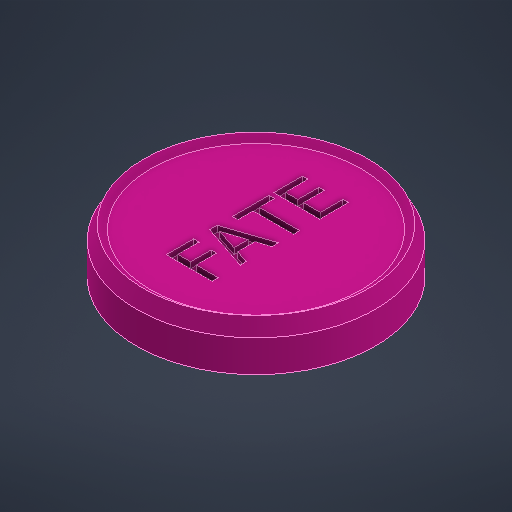
# Autodesk Inventor part: Fate Game Piece V1.01
Saved by Autodesk Inventor 2027 (Build 310192000, 192)
## iProperties
Created: 2025-10-12
Part Number: Fate Game Piece V1.01
Material: Generic
Document SubType Name: Modeling
Designer: Owner
Density: 1 g/cm^3
Appearance: Default
Author: Owner
Autodesk Inventor part; units mm, degrees
ref_plane "YZ Plane" through (0, 0, 0) normal (1, 0, 0) x (0, 1, 0)
ref_plane "XZ Plane" through (0, 0, 0) normal (0, 1, 0) x (-1, 0, 0)
ref_plane "XY Plane" through (0, 0, 0) normal (0, 0, 1) x (1, 0, 0)
sketch "Sketch1" plane through (0, 0, 0) normal (0, 0, 1) x (1, 0, 0)
  line L0 (-15.875, 0) -> (0, 0)
  line L1 (0, 0) -> (0, -4.2333)
  line L2 (0, -4.2333) -> (-15.875, -4.2333)
  line L3 (-15.875, -4.2333) -> (-15.875, 0)
  line L4 (0, -4.2333) -> (-13.97, -4.2333)
  line L5 (-13.97, -4.2333) -> (-13.97, -5.5033)
  line L6 (-13.97, -5.5033) -> (0, -5.5033)
  line L7 (0, -5.5033) -> (0, -4.2333)
  line L8 (-15.875, -4.2333) -> (-13.6299, -4.2333) construction
  line L9 (-15.875, 0) -> (-12.7, 0) construction
  line L10 (-13.97, 1.27) -> (0, 1.27)
  line L11 (0, 1.27) -> (0, 0)
  line L12 (0, 0) -> (-13.97, 0)
  line L13 (-13.97, 0) -> (-13.97, 1.27)
  line L14 (-15.875, 0) -> (-12.8362, 0) construction
  line L15 (-15.875, -4.2333) -> (-13.97, -5.5033)
  line L16 (-15.875, 0) -> (-14.9225, 1.905)
  line L17 (-14.9225, 1.905) -> (-13.97, 1.27)
  line L18 (-13.97, 0) -> (-15.875, 0)
  line L19 (0, -6.985) -> (0, 3.3867) projected
  point P0 (0, 0)
  point P1 (-13.97, 0.635)
  point P2 (0, 0.635)
  point P3 (-6.985, -4.2333)
  point P4 (-14.9225, 0)
  dimension "d0" = 0
  dimension "d1" = 4.2333
  dimension "d2" = 15.875
  dimension "d3" = 0
  dimension "d5" = 13.97
  dimension "d9" = 13.97
  dimension "d10" = 1.27
  dimension "d11" = 1.27
  dimension "d12" = 0.635
  dimension "d13" = 0
  constraints: 38 end point, 6 horizontal, 6 parallel, 4 midpoint, 3 perpendicular, 1 collinear
  measures "d0" distance from line of point (0, 0) L1
  measures "d1" distance between parallel lines of L2 L0
  measures "d2" distance of L1.end L2.end
  measures "d3" distance from line of point (0, 0) L0
  measures "d5" distance between parallel lines of L7 L5
  measures "d9" distance of point (-13.97, 0.635) point (0, 0.635)
  measures "d10" distance from line of L6 point (-6.985, -4.233)
  measures "d11" distance between parallel lines of L0 L10
  measures "d12" distance from line of L10 L16.end
  measures "d13" horizontal distance of L16.end point (-14.923, 0)
revolve "Revolution1" add sketch "Sketch1" angle 360 about axis through (0, -10, 0) along (0, 1, 0)
sketch "Sketch2" plane through (0, 1.27, 0) normal (0, 1, 0) x (1, 0, 0)
  line L0 (-2.3268, -5.2364) -> (-2.3268, -8.072)
  line L1 (-2.3268, -8.072) -> (-0.6076, -8.072)
  line L2 (-0.6076, -8.072) -> (-0.6076, -5.355)
  line L3 (-0.6076, -5.355) -> (0.1136, -5.355)
  line L4 (0.1136, -5.355) -> (0.1136, -8.072)
  line L5 (0.1136, -8.072) -> (3.048, -8.072)
  line L6 (3.048, -8.072) -> (3.048, -8.8822)
  line L7 (3.048, -8.8822) -> (-3.048, -8.8822)
  line L8 (-3.048, -8.8822) -> (-3.048, -5.2364)
  line L9 (-3.048, -5.2364) -> (-2.3268, -5.2364)
  line L10 (3.048, -5.1673) -> (-3.048, -3.1122)
  line L11 (-3.048, -3.1122) -> (-3.048, -2.1143)
  line L12 (-3.048, -2.1143) -> (3.048, -0.0593)
  line L13 (3.048, -0.0593) -> (3.048, -0.9139)
  line L14 (3.048, -0.9139) -> (1.3437, -1.4672)
  line L15 (1.3437, -1.4672) -> (1.3437, -3.7939)
  line L16 (1.3437, -3.7939) -> (3.048, -4.3472)
  line L17 (3.048, -4.3472) -> (3.048, -5.1673)
  line L18 (0.6521, -1.6895) -> (-2.2181, -2.633)
  line L19 (-2.2181, -2.633) -> (0.6521, -3.5716)
  line L20 (0.6521, -3.5716) -> (0.6521, -1.6895)
  line L21 (3.048, 1.9414) -> (-2.3268, 1.9414)
  line L22 (-2.3268, 1.9414) -> (-2.3268, -0.1037)
  line L23 (-2.3268, -0.1037) -> (-3.048, -0.1037)
  line L24 (-3.048, -0.1037) -> (-3.048, 4.7968)
  line L25 (-3.048, 4.7968) -> (-2.3268, 4.7968)
  line L26 (-2.3268, 4.7968) -> (-2.3268, 2.7516)
  line L27 (-2.3268, 2.7516) -> (3.048, 2.7516)
  line L28 (3.048, 2.7516) -> (3.048, 1.9414)
  line L29 (3.048, 5.4143) -> (-3.048, 5.4143)
  line L30 (-3.048, 5.4143) -> (-3.048, 9.228)
  line L31 (-3.048, 9.228) -> (-2.3268, 9.228)
  line L32 (-2.3268, 9.228) -> (-2.3268, 6.2244)
  line L33 (-2.3268, 6.2244) -> (-0.657, 6.2244)
  line L34 (-0.657, 6.2244) -> (-0.657, 9.0254)
  line L35 (-0.657, 9.0254) -> (0.0642, 9.0254)
  line L36 (0.0642, 9.0254) -> (0.0642, 6.2244)
  line L37 (0.0642, 6.2244) -> (2.3268, 6.2244)
  line L38 (2.3268, 6.2244) -> (2.3268, 9.228)
  line L39 (2.3268, 9.228) -> (3.048, 9.228)
  line L40 (3.048, 9.228) -> (3.048, 5.4143)
  point P0 (0, 0)
  point P1 (0, 0)
  constraints: 1 other
extrude "Extrusion1" cut sketch "Sketch2" against normal blind 0.7937
equation "\"d17\" = 0.5 * d16"
equation "\"d16\" = 12.7"
body "Solid1"
